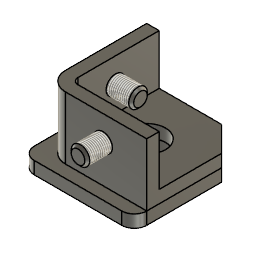
Aeolus Task 1 (Autodesk Fusion 360 design; units mm, degrees)
part number: 2026-09-11-14-58-28-559
part number: 2026-09-11-15-11-58-250
part number: 2026-09-11-15-12-00-316
part number: 2026-09-11-15-12-01-844
Autodesk Fusion 360 part; units mm, degrees
sketch "Sketch1" plane through (0, 0, 0) normal (0, 0, 1) x (1, 0, 0)
  line L0 (0, 0) -> (80, 0)
  line L1 (90, 10) -> (90, 80)
  line L2 (80, 90) -> (10, 90)
  line L3 (0, 80) -> (0, 0)
  line L4 (0, 20) -> (20, 0)
  circle A0 centre (40, 40) radius 17.5
  arc A1 (10, 90) -> (0, 80) centre (10, 80) ccw
  arc A2 (90, 80) -> (80, 90) centre (80, 80) ccw
  arc A3 (80, 0) -> (90, 10) centre (80, 10) ccw
  point P0 (90, 0)
  point P1 (0, 90)
  dimension "d1" = 90
  dimension "d2" = 90
  dimension "d3" = 20
  dimension "d4" = 20
  dimension "d5" = 35
  dimension "d6" = 40
  dimension "d7" = 40
  dimension "d8" = 10
  constraint horizontal L0
  constraint vertical L1
  constraint horizontal L2
  constraint vertical L3
  constraint coincident L0.start L3.end
  constraint coincident L3 L4.start
  constraint coincident L0 L4.end
  constraint coincident P1 L2
  constraint coincident P1 L3
  constraint tangent L2 A1
  constraint tangent L3 A1
  constraint tangent L1 A2
  constraint tangent L2 A2
  constraint equal A1 A2
  constraint coincident P0 L0
  constraint coincident P0 L1
  constraint tangent L0 A3
  constraint tangent L1 A3
  constraint equal A1 A3
  measures "d1" distance of L0.start P0
  measures "d2" distance of L0.start P1
  measures "d3" distance of L0.start L4.end
  measures "d4" distance of L0.start L4.start
  measures "d5" diameter of A0
  measures "d6" distance of L0 A0.centre
  measures "d7" distance of L3 A0.centre
  measures "d8" radius of A1
extrude "Extrude1" add sketch "Sketch1" along normal blind 10 contours L0 L1 L2 L3 L4 A1 A2 A3 makes body 1
sketch "Sketch2" plane through (0, 0, 0) normal (0, 0, 1) x (1, 0, 0)
  line L0 (0, 0) -> (80, 0)
  line L1 (80, 0) -> (80, 80)
  line L2 (80, 80) -> (0, 80)
  line L3 (0, 80) -> (0, 0)
  line L4 (0, 20) -> (20, 0)
  circle A0 centre (40, 40) radius 15
  dimension "d11" = 80
  dimension "d12" = 80
  dimension "d13" = 20
  dimension "d14" = 20
  dimension "d15" = 30
  dimension "d16" = 40
  dimension "d17" = 40
  constraint horizontal L0
  constraint vertical L1
  constraint horizontal L2
  constraint vertical L3
  constraint coincident L0.start L3.end
  constraint coincident L3 L4.start
  constraint coincident L0 L4.end
  measures "d11" distance of L0.start L0.end
  measures "d12" distance of L0.start L2.end
  measures "d13" distance of L0.start L4.end
  measures "d14" distance of L0.start L4.start
  measures "d15" diameter of A0
  measures "d16" distance of L3 A0.centre
  measures "d17" distance of L0 A0.centre
extrude "Extrude2" add sketch "Sketch2" along normal blind 10 separate body contours L0 L1 L2 L3 L4 makes body 2
sketch "Sketch3" plane through (0, 0, 10) normal (0, 0, 1) x (-1, 0, 0)
  circle A0 centre (-40, -40) radius 15
  line L0 (0, -20) -> (-20, 0)
  line L1 (-20, 0) -> (-80, 0)
  line L2 (-80, 0) -> (-80, -80)
  line L3 (-80, -80) -> (0, -80)
  line L4 (0, -80) -> (0, -20)
  line L5 (0, -80) -> (-90, -80)
  line L6 (-90, -80) -> (-90, -70)
  line L7 (-90, -70) -> (0, -70)
  line L8 (0, -70) -> (0, -80)
  line L9 (-80, -80) -> (-70, -80)
  line L10 (-70, -80) -> (-70, 0.2075)
  line L11 (-70, 0.2075) -> (-80, 0.2075)
  line L12 (-80, 0.2075) -> (-80, -80)
  dimension "d20" = 10
  dimension "d21" = 10
  constraint horizontal L5
  constraint vertical L6
  constraint horizontal L7
  constraint vertical L8
  constraint coincident L3.end L4.start
  constraint horizontal L9
  constraint vertical L10
  constraint horizontal L11
  constraint vertical L12
  constraint coincident L2.end L3.start
  measures "d20" distance of L3.end L7.end
  measures "d21" distance of L2.end L9.end
extrude "Extrude3" add sketch "Sketch3" along normal blind 40 contours L3 L4 L5 L7 L8 L10 | L1 L2 L7 L10 L12 | L2 L3 L5 L7 L9 L10 L12 bodies 2
fillet "Fillet1" radius 5 1 edges at (70, 70, 30) on bodies 2
fillet "Fillet2" radius 15 1 edges at (80, 80, 25) on bodies 2
sketch "Sketch4" plane through (0, 80, 0) normal (0, 1, 0) x (-1, 0, 0)
  line L0 (-65, 50) -> (-65, 0)
  line L1 (-65, 0) -> (0, 0)
  line L2 (0, 0) -> (0, 50)
  line L3 (0, 50) -> (-65, 50)
  circle A0 centre (-35, 30) radius 7.5
  line L4 (-20, 10) -> (-70, 10)
  dimension "d28" = 15
  dimension "d29" = 20
  dimension "d30" = 35
  measures "d28" diameter of A0
  measures "d29" distance of A0.centre L4
  measures "d30" distance of L2 A0.centre
extrude "Extrude4" cut sketch "Sketch4" against normal blind 20 contours A0 bodies 2
sketch "Sketch5" plane through (70, 0, 0) normal (-1, 0, 0) x (0, -1, 0)
  line L0 (-65, 50) -> (-65, 10)
  line L1 (-65, 10) -> (0, 10)
  line L2 (0, 10) -> (0, 50)
  line L3 (0, 50) -> (-65, 50)
  circle A0 centre (-35, 30) radius 7.5
  dimension "d33" = 15
  dimension "d34" = 20
  dimension "d35" = 35
  measures "d33" diameter of A0
  measures "d34" distance of L1 A0.centre
  measures "d35" distance of L2 A0.centre
extrude "Extrude5" cut sketch "Sketch5" against normal blind 30 contours A0 bodies 2
sketch "Sketch6" plane through (0, 0, 0) normal (0, 0, 1) x (1, 0, 0)
  circle A0 centre (0, 0) radius 7.5
  dimension "d38" = 15
  constraint coincident A0.centre origin
  measures "d38" diameter of A0
extrude "Extrude6" add sketch "Sketch6" along normal blind 30 separate body makes body 3
sketch "Sketch7" plane through (0, 0, 30) normal (0, 0, 1) x (-1, 0, 0)
  circle A0 centre (0, 0) radius 7.5
  circle A1 centre (0, 0) radius 12.5
  dimension "d41" = 25
  constraint coincident A0.centre A1.centre
  measures "d41" diameter of A1
extrude "Extrude7" add sketch "Sketch7" along normal blind 5 contours A0 | A1 bodies 3
chamfer "Chamfer1" distance 2 angle 45 2 edges at (11.6541, 4.5202, 35) (-6.9925, -2.7121, 0) tangent chain off on bodies 3
thread "Thread1" "ISO Metric profile 15.0 M15x1.5 M15x1.5 6g" major diameter 14.85 minor diameter 13.1369 pitch 1.5 angle 60 resizes the face on face at (7.4907, -0.3738, 20.6667) on bodies 3
sketch "Sketch8" plane through (0, 0, 35) normal (0, 0, 1) x (-1, 0, 0)
  circle A0 centre (0, 0) radius 10.5
  line L0 (2.8657, -4.0973) -> (4.9812, 0.4331)
  line L1 (4.9812, 0.4331) -> (2.1155, 4.5304)
  line L2 (2.1155, 4.5304) -> (-2.8657, 4.0973)
  line L3 (-2.8657, 4.0973) -> (-4.9812, -0.4331)
  line L4 (-4.9812, -0.4331) -> (-2.1155, -4.5304)
  line L5 (-2.1155, -4.5304) -> (2.8657, -4.0973)
  dimension "d47" = 5
  constraint coincident A0.centre origin
  measures "d47" distance of L0.start A0.centre
extrude "Extrude8" cut sketch "Sketch8" against normal blind 5 contours L0 L1 L2 L3 L4 L5 bodies 3
copy_body "Body->Comp1" bodies 3 removing the originals makes body 4 in component "Component"
copy_body "Body->Comp2" bodies 2 removing the originals makes body 5 in component "Component'"
copy_body "Body->Comp3" bodies 1 removing the originals makes body 6 in component "Component''"
move_body "Move1" bodies 5 to x (0, 0, 1) y (0, 1, 0) z (-1, 0, 0) at (90, 0, -90) in component "Component'"
move_body "Move1'" bodies 4 to x (0, 0, 1) y (0, 1, 0) z (-1, 0, 0) at (38.0986, 0, -38.0986) in component "Component"
move_body "Move1''" bodies 6 to x (0, 0, 1) y (0, 1, 0) z (-1, 0, 0) at (90, 0, -90) in component "Component''"
move_body "Move2" bodies 5 to x (0, 0, -1) y (0, 1, 0) z (1, 0, 0) at (100, 0, 80) in component "Component'"
move_body "Move2'" bodies 6 to x (0, 0, -1) y (0, 1, 0) z (1, 0, 0) at (100, 0, 80) in component "Component''"
component "Component" placed x (0, -1, 0) y (1, 0, 0) z (0, 0, 1) at (105, -80.8447, 0)
component "Component'" placed x (-1, 0, 0) y (0, -1, 0) z (0, 0, 1) at (150, -18.9433, -58.0986)
component "Component''" placed x (-1, 0, 0) y (0, -1, 0) z (0, 0, 1) at (150, -18.9433, -68.0986)
component "Component" placed x (1, 0, 0) y (0, 1, 0) z (0, 0, 1) at (51.9014, -53.9433, 0)
